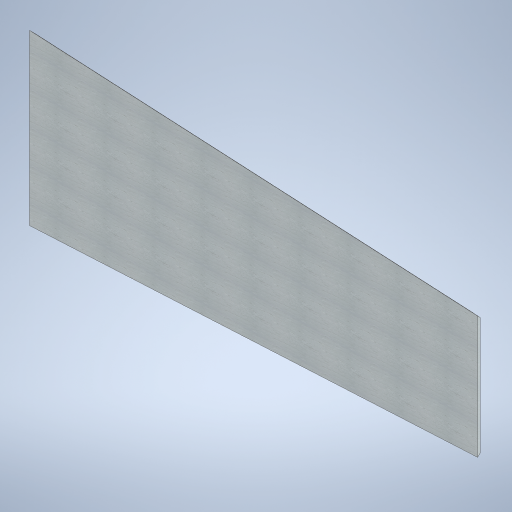
# Autodesk Inventor part: Wind Tunnel Output Body Single Panel
Saved by Autodesk Inventor 2023 (Build 270158000, 158)
## iProperties
Created: 2022-01-10
Part Number: Wind Tunnel Output Body Single Panel
Material: Wood (Oak)
Document SubType Name: Modeling
Designer: kamer
Density: 0.76 g/cm^3
Appearance: Wood - Painted White
Author: kamer
Autodesk Inventor part; units mm, degrees
ref_plane "YZ Plane" through (0, 0, 0) normal (1, 0, 0) x (0, 1, 0)
ref_plane "XY Plane" through (0, 0, 0) normal (0, 0, 1) x (1, 0, 0)
sketch "Sketch1" plane through (0, 0, 0) normal (0, 0, 1) x (1, 0, 0)
  line L0 (0, 0) -> (1219.2, 0)
  line L1 (1219.2, 0) -> (1219.2, 459.74)
  line L2 (1219.2, 459.74) -> (0, 459.74)
  line L3 (0, 459.74) -> (0, 0)
  line L4 (1219.2, 396.24) -> (1244.6, 396.24) construction
  line L5 (1244.6, 396.24) -> (1244.6, 63.5) construction
  line L6 (1244.6, 63.5) -> (1219.2, 63.5) construction
  line L7 (1219.2, 396.24) -> (0, 459.74)
  line L8 (1219.2, 63.5) -> (0, 0)
  dimension "d0" = 1219.2
  dimension "d1" = 459.74
  dimension "d2" = 25.4
  dimension "d3" = 332.74
  dimension "d4" = 63.5
  constraints: 18 end point, 3 perpendicular, 2 horizontal, 2 parallel, 2 point on line
  measures "d0" distance of L2.end L1.end
  measures "d1" distance of L1.end L0.end
  measures "d2" distance of L4.start L4.end
  measures "d3" distance of L4.end L5.end
  measures "d4" distance between parallel lines of L2 L4
extrude "Extrusion1" add sketch "Sketch1" along normal blind 12.7 contours L3 L7 L1 L8
sketch "Sketch2" plane through (1219.2, 63.5, 0) normal (1, 0, 0) x (0, 0, -1)
  line L0 (-12.7, 332.74) -> (-12.7, 396.24) projected
  line L1 (-12.7, 332.74) -> (0, 320.0577)
  line L2 (0, 0) -> (0, 332.74) projected
  line L3 (-12.7, 332.74) -> (5.248, 332.74) construction
  line L4 (0, 320.0577) -> (0, 332.74)
  line L5 (0, 332.74) -> (-12.7, 332.74)
  point P0 (0, -63.5)
  dimension "d7" = 44.96
  constraints: 8 end point, 1 collinear, 1 equal length, 1 horizontal, 1 perpendicular, 1 point on line
  measures "d7" angle of L1 L3
sketch "Sketch3" plane through (0, 0, 0) normal (-1, 0, 0) x (0, 0, 1)
  line L0 (12.7, 396.24) -> (12.7, 459.74) projected
  line L1 (12.7, 459.74) -> (0, 447.0577)
  line L2 (0, 396.24) -> (0, 459.74) projected
  line L3 (12.7, 459.74) -> (30.648, 459.74) construction
  line L4 (0, 459.74) -> (12.7, 459.74) projected
  line L5 (0, 447.0577) -> (0, 459.74)
  line L6 (0, 459.74) -> (12.7, 459.74)
  point P0 (0, 0)
  dimension "d8" = 135.04
  constraints: 8 end point, 1 collinear, 1 equal length, 1 horizontal, 1 perpendicular, 1 point on line
  measures "d8" angle of L1 L3
loft "Loft1" cut profiles "Sketch3", "Sketch2"
sketch "Sketch4" plane through (0, 0, 0) normal (-1, 0, 0) x (0, 0, 1)
  line L0 (12.7, 0) -> (12.7, 63.5) projected
  line L1 (12.7, 0) -> (0, 12.6823)
  line L2 (0, 0) -> (0, 63.5) projected
  line L3 (12.7, 0) -> (30.648, 0) construction
  line L4 (0, 12.6823) -> (0, 0)
  line L5 (12.7, 0) -> (0, 0)
  dimension "d13" = 135.04
  constraints: 8 end point, 1 equal length, 1 horizontal, 1 perpendicular, 1 point on line, 1 vertical
  measures "d13" angle of L3 L1
sketch "Sketch5" plane through (1219.2, 63.5, 12.7) normal (1, 0, 0) x (0, 0, -1)
  line L0 (12.7, 0) -> (0, 0) projected
  line L1 (0, 0) -> (12.7, 12.6823)
  line L2 (12.7, 383.5577) -> (12.7, -63.5) projected
  line L3 (0, 0) -> (17.948, 0) construction
  line L4 (12.7, 12.6823) -> (12.7, 0)
  line L5 (12.7, -63.5) -> (12.7, 0) projected
  line L6 (12.7, 0) -> (0, 0)
  dimension "d14" = 44.96
  constraints: 8 end point, 2 point on line, 1 equal length, 1 horizontal, 1 perpendicular
  measures "d14" angle of L3 L1
loft "Loft2" cut profiles "Sketch5", "Sketch4"
ref_plane "Center Plane" through (0, 228.6, 0) normal (0, 1, 0) x (-1, 0, 0)
sketch "Sketch6" plane through (0, 228.6, 0) normal (0, 1, 0) x (-1, 0, 0)
  line L0 (-1219.2, 12.7) -> (-1219.2, 0) projected
  line L1 (-1219.2, 0) -> (0, 0) projected
  line L2 (-1219.2, 12.7) -> (-1206.4827, 12.7) construction
  line L3 (-1219.2, 0) -> (-1218.5378, 12.7)
  line L4 (-1219.2, 0) -> (-1206.4827, 0) construction
  line L5 (0, 12.7) -> (-1219.2, 12.7) projected
  dimension "d26" = 87.015
  constraints: 6 end point, 2 horizontal, 1 equal length, 1 point on line
  measures "d26" angle of L4 L3
extrude "Extrusion2" cut sketch "Sketch6" against normal through all both and the other way through all
sketch "Sketch8" plane through (1218.5378, 63.4655, 12.7) normal (0.9986, 0, 0.0521) x (0.0521, 0, -0.9986)
  line L0 (12.7173, 12.7168) -> (0, 0) projected
  line L1 (12.7173, 12.7168) -> (12.7173, 320.0922) projected
  line L2 (0, 332.809) -> (12.7173, 320.0922) projected
  line L3 (0, 0) -> (0, 332.809) projected
  line L4 (12.7173, 12.7168) -> (12.7173, 320.0922) projected
  line L5 (12.7173, 345.4922) -> (6.9515, 345.4922)
  line L6 (6.9515, 345.4922) -> (6.9515, -12.6832)
  line L7 (6.9515, -12.6832) -> (12.7173, -12.6832)
  line L8 (12.7173, -12.6832) -> (12.7173, 345.4922)
  point P0 (-50.772, -63.4655)
  dimension "d27" = 5.7658
  dimension "d28" = 25.4
  dimension "d29" = 25.4
  constraints: 8 end point, 2 parallel, 1 horizontal, 1 perpendicular, 1 point on line
  measures "d27" distance between parallel lines of L6 L1
  measures "d28" distance from line of L1.end L5
  measures "d29" distance from line of L0.start L7
extrude "Extrusion3" cut sketch "Sketch8" against normal blind 25.4 contours L8 L7 L6 L0 | L0 L6 L2 L1 | L2 L6 L5 L8
sketch "Sketch9" plane through (0, 228.6, 0) normal (0, 1, 0) x (-1, 0, 0)
  line L0 (-1193.5342, 4.4353) -> (-1193.7655, 0) projected
  line L1 (0, 0) -> (-1193.7655, 0) projected
  line L2 (0, 12.7) -> (0, 0) projected
  line L3 (-1218.5378, 12.7) -> (0, 12.7) projected
  line L4 (-1218.5378, 12.7) -> (-1218.8997, 5.758) projected
  line L5 (-1218.8997, 5.758) -> (-1193.5342, 4.4353) projected
  line L6 (0, 12.7) -> (-0.6622, 0)
  line L7 (0, 12.7) -> (12.7173, 12.7) construction
  point P0 (0, 0)
  dimension "d32" = 92.985
  constraints: 4 end point, 1 equal length, 1 horizontal, 1 point on line
  measures "d32" angle of L6 L7
extrude "Extrusion4" cut sketch "Sketch9" against normal through all both and the other way through all contours L6 L2 L1
body "Solid1"
